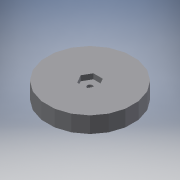
# Autodesk Inventor part: PropellerHub
Saved by Autodesk Inventor 2017 (Build 210142000, 142)
## iProperties
Created: 2017-08-04
Part Number: PropellerHub
Material: Generic
Document SubType Name: Modeling
Designer: vmiguel
Density: 1 g/cm^3
Appearance: Default
Author: vmiguel
Autodesk Inventor part; units mm, degrees
ref_plane "YZ Plane" through (0, 0, 0) normal (1, 0, 0) x (0, 1, 0)
ref_plane "XZ Plane" through (0, 0, 0) normal (0, 1, 0) x (-1, 0, 0)
ref_plane "XY Plane" through (0, 0, 0) normal (0, 0, 1) x (1, 0, 0)
sketch "Sketch2" plane through (0, 0, 0) normal (0, 0, 1) x (1, 0, 0)
  line L0 (20.59, 130) -> (59.7544, 117.2747)
  line L1 (59.7544, 117.2747) -> (93.0697, 93.0697)
  line L2 (93.0697, 93.0697) -> (117.2747, 59.7544)
  line L3 (117.2747, 59.7544) -> (130, 20.59)
  line L4 (130, 20.59) -> (130, -20.59)
  line L5 (130, -20.59) -> (117.2747, -59.7544)
  line L6 (117.2747, -59.7544) -> (93.0697, -93.0697)
  line L7 (93.0697, -93.0697) -> (59.7544, -117.2747)
  line L8 (59.7544, -117.2747) -> (20.59, -130)
  line L9 (20.59, -130) -> (-20.59, -130)
  line L10 (-20.59, -130) -> (-59.7544, -117.2747)
  line L11 (-59.7544, -117.2747) -> (-93.0697, -93.0697)
  line L12 (-93.0697, -93.0697) -> (-117.2747, -59.7544)
  line L13 (-117.2747, -59.7544) -> (-130, -20.59)
  line L14 (-130, -20.59) -> (-130, 20.59)
  line L15 (-130, 20.59) -> (-117.2747, 59.7544)
  line L16 (-117.2747, 59.7544) -> (-93.0697, 93.0697)
  line L17 (-93.0697, 93.0697) -> (-59.7544, 117.2747)
  line L18 (-59.7544, 117.2747) -> (-20.59, 130)
  line L19 (-20.59, 130) -> (20.59, 130)
  circle A0 centre (0, 0) radius 8
  point P0 (0, 130)
  dimension "d0" = 260
  dimension "d3" = 16
  constraints: 40 end point, 2 coincident, 1 centre point, 1 midpoint, 1 vertical alignment, 41 other
  measures "d0" distance between parallel lines of L9 L19
  measures "d3" diameter of A0
extrude "Extrusion1" add sketch "Sketch2" along normal blind 50
sketch "Sketch3" plane through (0, 0, 50) normal (0, 0, 1) x (1, 0, 0)
  circle A0 centre (0, 0) radius 8 projected
  line L0 (14.4338, 25) -> (28.8675, 0)
  line L1 (28.8675, 0) -> (14.4338, -25)
  line L2 (14.4338, -25) -> (-14.4338, -25)
  line L3 (-14.4338, -25) -> (-28.8675, 0)
  line L4 (-28.8675, 0) -> (-14.4338, 25)
  line L5 (-14.4338, 25) -> (14.4338, 25)
  point P0 (0, 25)
  dimension "d4" = 50
  constraints: 12 end point, 1 coincident, 1 midpoint, 1 vertical alignment, 13 other
  measures "d4" distance between parallel lines of L2 L5
extrude "Extrusion2" cut sketch "Sketch3" against normal blind 16
body "Solid1"
